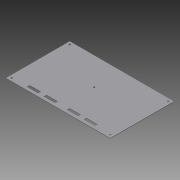
# Autodesk Inventor part: bottom_plate
Saved by Autodesk Inventor 2015 SP1 (Build 190203100, 203)
## iProperties
Created: 2016-08-02
Part Number: bottom_plate
Material: Generic
Document SubType Name: Modeling
Designer: polidorop
Density: 1 g/cm^3
Appearance: Default
Author: polidorop
Autodesk Inventor part; units mm, degrees
ref_plane "YZ Plane" through (0, 0, 0) normal (1, 0, 0) x (0, 1, 0)
ref_plane "XZ Plane" through (0, 0, 0) normal (0, 1, 0) x (-1, 0, 0)
ref_plane "XY Plane" through (0, 0, 0) normal (0, 0, 1) x (1, 0, 0)
sketch "Sketch2" plane through (0, 0, 0) normal (0, 0, 1) x (1, 0, 0)
  circle A0 centre (175, 88) radius 3.2
  circle A1 centre (175, -118) radius 3.2
  circle A2 centre (-175, -118) radius 3.2
  circle A3 centre (-175, 88) radius 3.2
  line L0 (-185, 98) -> (185, 98)
  line L1 (185, 98) -> (185, -128)
  line L2 (185, -128) -> (-185, -128)
  line L3 (-185, -128) -> (-185, 98)
  line L4 (-121, -108) -> (-81, -108)
  line L5 (-81, -108) -> (-81, -118.5)
  line L6 (-81, -118.5) -> (-121, -118.5)
  line L7 (-121, -118.5) -> (-121, -108)
  line L8 (-61, -108) -> (-21, -108)
  line L9 (-21, -108) -> (-21, -118.5)
  line L10 (-21, -118.5) -> (-61, -118.5)
  line L11 (-61, -118.5) -> (-61, -108)
  line L12 (21, -108) -> (61, -108)
  line L13 (61, -108) -> (61, -118.5)
  line L14 (61, -118.5) -> (21, -118.5)
  line L15 (21, -118.5) -> (21, -108)
  line L16 (81, -108) -> (121, -108)
  line L17 (121, -108) -> (121, -118.5)
  line L18 (121, -118.5) -> (81, -118.5)
  line L19 (81, -118.5) -> (81, -108)
  circle A4 centre (0, 0) radius 3.2
  constraints: 40 end point, 10 perpendicular, 6 parallel, 5 centre point, 4 equal radius, 3 collinear
extrude "Extrusion2" add sketch "Sketch2" along normal mid plane 2
body "Solid2"
